Autodesk Inventor part; units mm, degrees
(part 5 of 5)
sketch "Эскиз48" plane through (1.5, -2, 18) normal (0, 0, 1) x (1, 0, 0)
  line L0 (0, 377) -> (-1.5, 377) projected
  line L1 (-17, 372.5031) -> (0, 323.3605)
  line L2 (0, 374) -> (0, 0) projected
  point P0 (-1.5, 2)
  dimension "d258" = 52
  dimension "d259" = 17
  constraints: 2 end point
  measures "d258" distance of L1.start L1.end
  measures "d259" distance from line of L1.start L2
equation "\"d99\" = d97"
